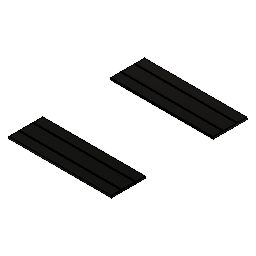
_6-9 (Long Straight).1fa60582-16a2-4a24-9422-7d1a460f0ce0 (Autodesk Fusion 360 design; units mm, degrees)
Autodesk Fusion 360 part; units mm, degrees
sketch "Sketch1" plane through (0, 0, 0) normal (0, 0, 1) x (1, 0, 0)
  line L0 (0, 0) -> (0, -812.8)
  line L1 (0, -812.8) -> (0, -2413)
  line L2 (0, -2413) -> (0, -3225.8)
  line L3 (0, 0) -> (1219.2, 0)
  line L4 (1219.2, 0) -> (0, 0)
  line L5 (0, 0) -> (0, -812.8)
  line L6 (0, -812.8) -> (1219.2, -812.8)
  line L7 (1219.2, -812.8) -> (1219.2, 0)
  line L8 (0, -3225.8) -> (1219.2, -3225.8)
  line L9 (1219.2, -3225.8) -> (0, -3225.8)
  line L10 (0, -3225.8) -> (0, -2413)
  line L11 (0, -2413) -> (1219.2, -2413)
  line L12 (1219.2, -2413) -> (1219.2, -3225.8)
  line L13 (1219.2, -812.8) -> (1219.2, 0)
  line L14 (1219.2, 0) -> (2438.4, 0)
  line L15 (2438.4, 0) -> (2438.4, -812.8)
  line L16 (2438.4, -812.8) -> (1219.2, -812.8)
  line L17 (1219.2, -3225.8) -> (1219.2, -2413)
  line L18 (1219.2, -2413) -> (2438.4, -2413)
  line L19 (2438.4, -2413) -> (2438.4, -3225.8)
  line L20 (2438.4, -3225.8) -> (1219.2, -3225.8)
  dimension "d1" = 812.8
  dimension "d2" = 1600.2
  dimension "d3" = 812.8
  dimension "d4" = 1219.2
  dimension "d5" = 1219.2
  dimension "d8" = 1219.2
  dimension "d9" = 1219.2
  constraint coincident L0.start L3.start
  constraint vertical L0
  constraint parallel L0 L1
  constraint parallel L1 L2
  constraint perpendicular L0 L3
  constraint horizontal L4
  constraint vertical L5
  constraint horizontal L6
  constraint vertical L7
  constraint perpendicular L2 L8
  constraint horizontal L9
  constraint vertical L10
  constraint horizontal L11
  constraint vertical L12
  constraint perpendicular L13 L14
  constraint parallel L13 L15
  constraint parallel L14 L16
  constraint perpendicular L17 L18
  constraint parallel L17 L19
  constraint parallel L18 L20
  measures "d1" distance of L0.start L0.end
  measures "d2" distance of L0.end L1.end
  measures "d3" distance of L1.end L2.end
  measures "d4" distance of L0.start L3.end
  measures "d5" distance of L2.end L8.end
  measures "d8" distance of L6.end L15.end
  measures "d9" distance of L8.end L19.end
extrude "Extrude2" add sketch "Sketch1" along normal blind 50.8 makes body 1 at (812.8, -270.9333, 0) makes body 2 at (812.8, -2954.8667, 0)
sketch "Sketch2" plane through (0, 0, 50.8) normal (0, 0, 1) x (-1, 0, 0)
  line L0 (-2438.4, 0) -> (0, 0)
  line L1 (0, 0) -> (0, 812.8)
  line L2 (0, 812.8) -> (-2438.4, 812.8)
  line L3 (-2438.4, 812.8) -> (-2438.4, 0)
  line L4 (-2438.4, 250.825) -> (0, 250.825)
  line L5 (-2438.4, 231.775) -> (0, 231.775)
  line L6 (0, 561.975) -> (-2438.4, 561.975)
  line L7 (0, 581.025) -> (-2438.4, 581.025)
  dimension "d12" = -250.825
  dimension "d13" = -231.775
  dimension "d14" = -250.825
  dimension "d15" = -231.775
extrude "Extrude3" add sketch "Sketch2" along normal blind 0.0279 contours L1 L3 L4 L5 | L1 L3 L6 L7 bodies 1
sketch "Sketch3" plane through (0, 0, 50.8) normal (0, 0, 1) x (-1, 0, 0)
  line L0 (-2438.4, 3225.8) -> (-2438.4, 2413)
  line L1 (-2438.4, 2413) -> (0, 2413)
  line L2 (0, 2413) -> (0, 3225.8)
  line L3 (0, 3225.8) -> (-2438.4, 3225.8)
  line L4 (-2438.4, 2663.825) -> (0, 2663.825)
  line L5 (-2438.4, 2644.775) -> (0, 2644.775)
  line L6 (0, 2974.975) -> (-2438.4, 2974.975)
  line L7 (0, 2994.025) -> (-2438.4, 2994.025)
  dimension "d18" = -250.825
  dimension "d19" = -231.775
  dimension "d20" = -250.825
  dimension "d21" = -231.775
extrude "Extrude4" add sketch "Sketch3" along normal blind 0.0279 contours L0 L2 L6 L7 | L0 L2 L4 L5 bodies 2
equation "d4 = ( 24 * 2 ) * 1 in"
equation "d5 = ( 24 * 2 ) * 1 in"
equation "d8 = ( 24 * 2 ) * 1 in"
equation "d9 = ( 24 * 2 ) * 1 in"
